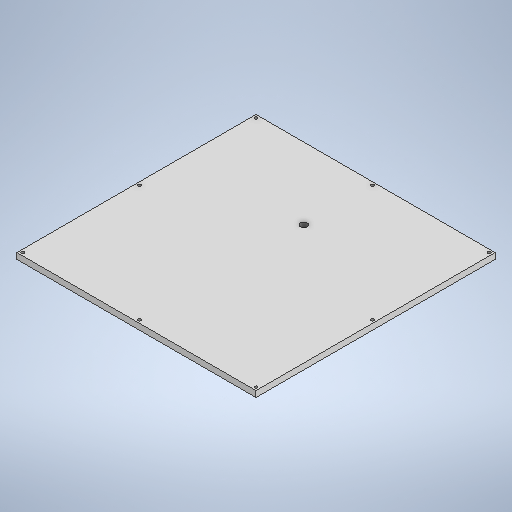
# Autodesk Inventor part: chassis_haut
Saved by Autodesk Inventor 2025.2 (Build 292293000, 293)
## iProperties
Created: 2026-03-16
Part Number: chassis_haut
Material: Générique
Document SubType Name: Modeling
Designer: genon
Density: 1 g/cm^3
Appearance: Par défaut
Author: genon
Autodesk Inventor part; units mm, degrees
ref_plane "YZ Plane" through (0, 0, 0) normal (1, 0, 0) x (0, 1, 0)
ref_plane "XZ Plane" through (0, 0, 0) normal (0, 1, 0) x (-1, 0, 0)
ref_plane "XY Plane" through (0, 0, 0) normal (0, 0, 1) x (1, 0, 0)
sketch "Esquisse1" plane through (0, 0, 0) normal (0, 1, 0) x (-1, 0, 0)
  line L0 (-100, 100) -> (100, 100)
  line L1 (100, 100) -> (100, -100)
  line L2 (100, -100) -> (-100, -100)
  line L3 (-100, -100) -> (-100, 100)
  line L4 (-100, 100) -> (100, -100) construction
  line L5 (100, 100) -> (-100, -100) construction
  point P0 (0, 0)
  dimension "d0" = 200
  dimension "d1" = 200
  constraints: 12 end point, 2 midpoint, 2 parallel, 1 horizontal, 1 perpendicular
  measures "d0" distance of L1.end L2.end
  measures "d1" distance of L0.end L1.end
extrude "Extrusion1" add sketch "Esquisse1" along normal blind 5
sketch "Esquisse2" plane through (0, 5, 0) normal (0, 1, 0) x (1, 0, 0)
  line L0 (0, 0) -> (0, -97.5)
  line L1 (0, -97.5) -> (-97.5, -97.5)
  line L2 (0, 0) -> (-32.0024, 0)
  point P0 (97.5, -97.5)
  point P1 (-97.5, 97.5)
  point P2 (97.5, 97.5)
  dimension "d4" = 97.5
  dimension "d5" = 97.5
  constraints: 6 end point, 3 symmetric about line, 1 coincident, 1 horizontal, 1 perpendicular, 1 vertical
  measures "d4" distance of L0.start L0.end
  measures "d5" distance of L0.end L1.end
hole "Perçage1" at (-97.5, 5, 97.5) at (97.5, 5, 97.5) at (-97.5, 5, -97.5) at (97.5, 5, -97.5) direction (0, -1, 0) diameter 2.459 end through all thread size "M3x0.5" class "6H" standard "ISO Metric profile"
sketch "Esquisse3" plane through (0, 5, 0) normal (0, 1, 0) x (1, 0, 0)
  line L0 (0, 0) -> (-97.5, 0)
  line L1 (0, 0) -> (0, 97.5)
  point P0 (97.5, 0)
  point P1 (0, -97.5)
  dimension "d13" = 97.5
  dimension "d14" = 97.5
  constraints: 4 end point, 2 coincident, 2 symmetric about line, 1 horizontal, 1 vertical
  measures "d13" distance of L0.start L0.end
  measures "d14" distance of L0.start L1.end
hole "Perçage2" at (-97.5, 5, 0) at (0, 5, -97.5) at (97.5, 5, 0) at (0, 5, 97.5) direction (0, -1, 0) diameter 2.459 end through all thread size "M3x0.5" class "6H" standard "ISO Metric profile"
sketch "Esquisse4" plane through (0, 5, 0) normal (0, 1, 0) x (1, 0, 0)
  line L0 (0, 0) -> (0, 40)
  dimension "d22" = 40
  constraints: 2 end point, 1 coincident, 1 vertical
  measures "d22" distance of L0.start L0.end
hole "Perçage3" at (0, 5, -40) direction (0, -1, 0) diameter 5.9175 end through all thread size "M7x1" class "6H" standard "ISO Metric profile"
